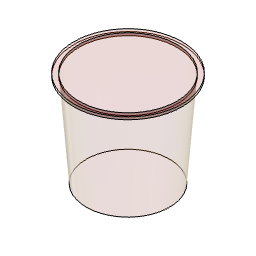
Tower 80mm (Autodesk Fusion 360 archive; units mm, degrees)
design "Jiffy Pot Mockup"
Autodesk Fusion 360 part; units mm, degrees
sketch "Sketch1" plane through (0, 0, 0) normal (0, 0, 1) x (1, 0, 0)
  circle A0 centre (0, 0) radius 33.5
  dimension "d1" = 67
  constraint coincident A0.centre origin
  measures "d1" diameter of A0
ref_plane "WorkPlane1" through (0, 0, 77) normal (0, 0, 1) x (1, 0, 0)
sketch "Sketch2" plane through (0, 0, 77) normal (0, 0, 1) x (1, 0, 0)
  circle A0 centre (0, 0) radius 39.5
  dimension "d3" = 79
  constraint coincident A0.centre origin
  measures "d3" diameter of A0
loft "Loft1" add profiles "Sketch1", "Sketch2" section 1 section 2
sketch "Sketch3" plane through (0, 0, 77) normal (0, 0, 1) x (-1, 0, 0)
  circle A0 centre (0, 0) radius 39.5
  circle A1 centre (0, 0) radius 43.5
  dimension "d4" = 87
  constraint coincident A0.centre A1.centre
  measures "d4" diameter of A1
extrude "Extrude1" add sketch "Sketch3" against normal blind 2
